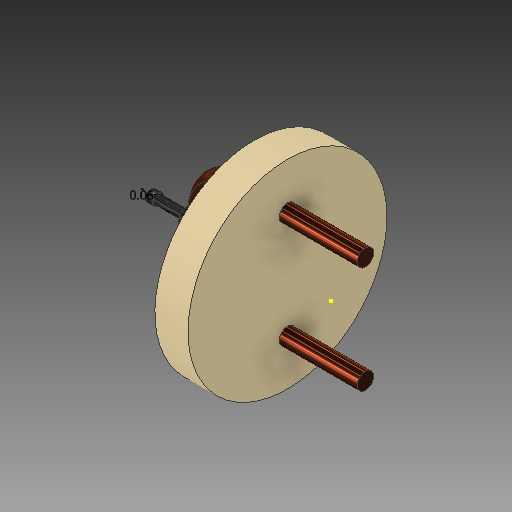
# Autodesk Inventor part: Cathode
Saved by Autodesk Inventor 2017.3 (Build 213256000, 256)
## iProperties
Created: 2017-02-04
Part Number: Cathode
Material: Generic
Document SubType Name: Modeling
Designer: Mac
Density: 1 g/cm^3
Appearance: Default
Author: Mac
Autodesk Inventor part; units mm, degrees
ref_plane "YZ Plane" through (0, 0, 0) normal (1, 0, 0) x (0, 1, 0)
ref_plane "XZ Plane" through (0, 0, 0) normal (0, 1, 0) x (-1, 0, 0)
ref_plane "XY Plane" through (0, 0, 0) normal (0, 0, 1) x (1, 0, 0)
sketch "Sketch1" plane through (0, 0, 0) normal (1, 0, 0) x (0, 1, 0)
  circle A0 centre (0, 0) radius 6
  dimension "d0" = 12
  constraints: 1 centre point, 1 coincident
  measures "d0" diameter of A0
extrude "Extrusion1" add sketch "Sketch1" along normal blind 2
sketch "Sketch2" plane through (2, 0, 0) normal (1, 0, 0) x (0, 0, -1)
  line L0 (0.5, 3.725) -> (-0.5, 3.725)
  line L1 (-0.5, 3.725) -> (-0.5, -3.725)
  line L2 (-0.5, -3.725) -> (0.5, -3.725)
  line L3 (0.5, -3.725) -> (0.5, 3.725)
  circle A0 centre (0, 3.225) radius 0.5
  circle A1 centre (0, -3.225) radius 0.5
  point P0 (0, 0)
  dimension "d3" = 1
  dimension "d4" = 7.45
  dimension "d5" = 1
  dimension "d6" = 1
  constraints: 8 end point, 2 centre point, 2 coincident, 2 parallel, 1 horizontal, 1 perpendicular
  measures "d3" distance of L2.end L1.end
  measures "d4" distance of L1.end L0.end
  measures "d5" diameter of A0
  measures "d6" diameter of A1
move or copy body "Move Body1" bodies to move or copy 1 copy no translate (-4.7, 0, 0)
extrude "Extrusion2" add sketch "Sketch2" against normal blind 7.7 contours A0 | A1
ref_plane "Work Plane2" through (-8.2, 0, 0) normal (-1, 0, 0) x (0, 0, 1)
sketch "Sketch3" plane through (-5.7, 3.225, 0) normal (-1, 0, 0) x (0, 0, 1)
  circle A0 centre (0, 0) radius 0.5
  point P0 (0, -3.225)
  dimension "d14" = 1
  constraints: 1 centre point
  measures "d14" diameter of A0
sketch "Sketch4" plane through (-8.2, 0, 0) normal (-1, 0, 0) x (0, 0, 1)
  point P0 (0, 0)
sketch "Sketch5" plane through (-8.2, 0, 0) normal (-1, 0, 0) x (0, 0, 1)
  point P0 (0, 0)
  point P1 (0, 1.225)
sketch "Sketch6" plane through (0, 0, 0) normal (0, 0, 1) x (1, 0, 0)
  line L0 (-5.7, 3.725) -> (-5.7, 2.725) projected
  arc A0 (-5.7, 3.225) -> (-8.1807, 1.2453) centre (-5.8485, 0.867) ccw
  point P0 (0, 0)
  constraints: 2 point on circle, 1 centre point, 1 midpoint
sweep "Sweep1" add profiles "Sketch3" path "Sketch6" keep normal constant yes path curves A0
sketch "Sketch7" plane through (-5.7, -3.225, 0) normal (-1, 0, 0) x (0, 0, 1)
  circle A0 centre (0, 0) radius 0.5
  point P0 (0, 3.225)
  constraints: 1 centre point
sketch "Sketch8" plane through (-8.2, 0, 0) normal (-1, 0, 0) x (0, 0, 1)
  point P0 (0, 0)
  point P1 (0, -1.225)
sketch "Sketch9" plane through (0, 0, 0) normal (0, 0, 1) x (1, 0, 0)
  line L0 (-5.7, -2.725) -> (-5.7, -3.725) projected
  arc A0 (-8.2009, -1.2247) -> (-5.7, -3.225) centre (-5.8008, -0.7875) ccw
  point P0 (0, 0)
  constraints: 2 point on circle, 1 centre point, 1 midpoint
ref_plane "Work Plane3" through (-8.2009, -1.2247, 0) normal (-1, 0, 0) x (0, 0, 1)
sweep "Sweep2" add profiles "Sketch7" path "Sketch9" keep normal constant yes path curves A0
ref_plane "Work Plane4" through (-8.2, -1.225, 0) normal (0, 0, 1) x (0, 1, 0)
ref_plane "Work Plane5" through (-8.2, -1.225, 0.5) normal (0, 0, 1) x (0, 1, 0)
ref_plane "Work Plane6" through (-8.2, -1.225, -0.5) normal (0, 0, 1) x (0, 1, 0)
sketch "Sketch10" plane through (-8.2, -1.225, 0.5) normal (0, 0, 1) x (0, 1, 0)
  line L0 (-0.9711, -0.541) -> (0.5671, -0.541)
  line L1 (0.5671, -0.541) -> (0.5671, 0.0009)
  line L2 (0.5671, 0.0009) -> (-0.9711, 0.0009)
  line L3 (-0.9711, 0.0009) -> (-0.9711, -0.541)
  point P0 (1.225, -8.2)
  constraints: 8 end point, 2 parallel, 1 horizontal, 1 perpendicular
extrude "Extrusion3" add sketch "Sketch10" along normal blind 0.2
sketch "Sketch11" plane through (-8.2, -1.225, 0) normal (0, 0, 1) x (0, 1, 0)
  line L0 (0.5671, -0.541) -> (0.5671, 0.0009) projected
  line L1 (0.5671, -0.541) -> (1.8594, -0.541)
  line L2 (1.8594, -0.541) -> (1.8594, 0.0009)
  line L3 (1.8594, 0.0009) -> (0.5671, 0.0009)
  line L4 (0.5671, 0.0009) -> (0.5671, -0.541)
  point P0 (1.225, -8.2)
  constraints: 8 end point, 2 parallel, 1 horizontal, 1 perpendicular
extrude "Extrusion4" add sketch "Sketch11" along normal blind 0.1
sketch "Sketch12" plane through (-8.2, -1.225, -0.5) normal (0, 0, 1) x (0, 1, 0)
  line L0 (0.5671, -0.541) -> (1.8594, -0.541) projected
  line L1 (1.8594, -0.541) -> (3.395, -0.541)
  line L2 (3.395, -0.541) -> (3.395, -0.0193)
  line L3 (3.395, -0.0193) -> (1.8594, -0.0193)
  line L4 (1.8594, -0.0193) -> (1.8594, -0.541)
  point P0 (1.225, -8.2)
  constraints: 8 end point, 2 parallel, 1 horizontal, 1 perpendicular
extrude "Extrusion5" add sketch "Sketch12" against normal blind 0.2
sketch "Sketch13" plane through (-8.2, -1.225, 0) normal (0, 0, -1) x (-1, 0, 0)
  line L0 (-0.541, 0.5671) -> (0.0009, 0.5671) projected
  line L1 (-0.541, 3.395) -> (-0.541, 1.8594) projected
  line L2 (0.0009, 0.5671) -> (-0.541, 0.5671)
  line L3 (-0.541, 0.5671) -> (-0.541, 1.8594)
  line L4 (-0.541, 1.8594) -> (0.0009, 1.8594)
  line L5 (0.0009, 1.8594) -> (0.0009, 0.5671)
  point P0 (-8.2, 1.225)
  constraints: 8 end point, 2 parallel, 1 horizontal, 1 perpendicular
extrude "Extrusion6" add sketch "Sketch13" along normal blind 0.1
sketch "Sketch14" plane through (-8.2, -1.225, 0.1) normal (0, 0, 1) x (1, 0, 0)
  point P0 (8.2, 1.225)
sketch "Sketch15" plane through (-8.2, -1.225, 0.1) normal (0, 0, 1) x (1, 0, 0)
  line L0 (-0.0009, 1.8594) -> (-0.0009, 0.5671) projected
  line L1 (-0.0009, 0.5896) -> (-0.0009, 0.8396)
  point P0 (8.2, 1.225)
  constraints: 2 end point, 1 point on line
sketch "Sketch16" plane through (-8.2, -1.225, 0.1) normal (0, 0, 1) x (1, 0, 0)
  line L0 (0.541, 1.8594) -> (0.541, 0.5671) projected
  line L1 (-0.0009, 1.8594) -> (-0.0009, 0.5671) projected
  line L2 (0.541, 0.5671) -> (-0.0009, 0.5671)
  line L3 (-0.0009, 0.5671) -> (-0.0009, 0.8171)
  line L4 (-0.0009, 0.8171) -> (0.541, 0.8171)
  line L5 (0.541, 0.8171) -> (0.541, 0.5671)
  point P0 (8.2, 1.225)
  dimension "d33" = 0.25
  constraints: 8 end point, 2 parallel, 1 horizontal, 1 perpendicular, 1 point on line
  measures "d33" distance of L2.end L3.end
extrude "Extrusion7" add sketch "Sketch16" along normal blind 0.6
sketch "Sketch17" plane through (-8.2, -1.225, -0.1) normal (0, 0, -1) x (-1, 0, 0)
  line L0 (0.0009, 1.8594) -> (0.0009, 0.8171) projected
  line L1 (-0.541, 0.8171) -> (-0.541, 1.8594) projected
  line L2 (0.0009, 1.8594) -> (-0.541, 1.8594)
  line L3 (-0.541, 1.8594) -> (-0.541, 1.6094)
  line L4 (-0.541, 1.6094) -> (0.0009, 1.6094)
  line L5 (0.0009, 1.6094) -> (0.0009, 1.8594)
  point P0 (-8.2, 1.225)
  dimension "d36" = 0.25
  constraints: 8 end point, 2 parallel, 1 horizontal, 1 perpendicular, 1 point on line
  measures "d36" distance of L3.end L2.end
extrude "Extrusion8" add sketch "Sketch17" along normal blind 0.6
sketch "Sketch18" plane through (-8.1807, 1.2453, -0.5) normal (-1, 0, 0) x (0, 0, 1)
  line L0 (0, 0) -> (0, -0.6109) projected
  line L1 (0, 0.9247) -> (-0.2, 0.9247) projected
  line L2 (0, -0.6109) -> (-0.2, -0.6109)
  line L3 (-0.2, -0.6109) -> (-0.2, 0.9247)
  line L4 (-0.2, 0.9247) -> (0, 0.9247)
  line L5 (0, 0.9247) -> (0, -0.6109)
  point P0 (0.5, -1.2453)
  constraints: 8 end point, 2 parallel, 1 horizontal, 1 perpendicular
extrude "Extrusion9" add sketch "Sketch18" along normal blind 0.02
ref_plane "Work Plane7" through (-8.1908, -1.2247, 0) normal (-1, 0, 0) x (0, 0, 1)
sketch "Sketch19" plane through (-8.1908, -1.2247, 0) normal (-1, 0, 0) x (0, 0, 1)
  circle A0 centre (0, 1.2247) radius 0.55
  dimension "d41" = 1.1
  constraints: 1 centre point, 1 coincident
  measures "d41" diameter of A0
extrude "Extrusion10" add sketch "Sketch19" along normal mid plane 1.064
sketch "Sketch20" plane through (-8.7228, 0, 0) normal (-1, 0, 0) x (0, 0, 1)
  circle A0 centre (0, 0) radius 0.275
  dimension "d44" = 0.55
  constraints: 1 centre point, 1 coincident
  measures "d44" diameter of A0
extrude "Extrusion11" add sketch "Sketch20" along normal blind 1.8
sketch "Sketch21" plane through (-10.5228, 0, 0) normal (-1, 0, 0) x (0, 0, 1)
  circle A0 centre (0, 0) radius 0.35
  dimension "d47" = 0.7
  constraints: 1 centre point, 1 coincident
  measures "d47" diameter of A0
extrude "Extrusion12" add sketch "Sketch21" along normal blind 0.4
ref_plane "Work Plane9" through (-11.1228, 0, 0) normal (-1, 0, 0) x (0, 0, 1)
ref_plane "Work Plane8" through (-11.1998, 0, 0) normal (-1, 0, 0) x (0, 0, 1)
sketch "Sketch22" plane through (-11.1228, 0, 0) normal (-1, 0, 0) x (0, 0, 1)
  circle A0 centre (0, 0) radius 0.03
  dimension "d52" = 0.06
  constraints: 1 centre point, 1 coincident
  measures "d52" diameter of A0
sketch "Sketch23" plane through (-11.1998, 0, 0) normal (-1, 0, 0) x (0, 0, 1)
  point P0 (0, 0)
  point P1 (0, 0)
  constraints: 1 coincident
loft "Loft1" add section 1 edges at (-10.9228, 0, -0.35) section 2 point at (-11.1998, 0, 0)
body "Solid1"
